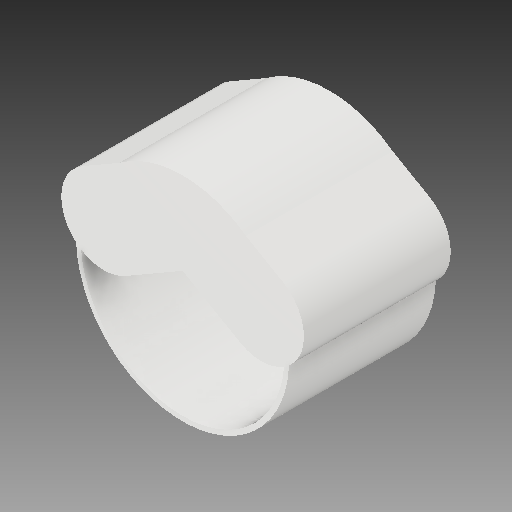
# Autodesk Inventor part: BA001
Saved by Autodesk Inventor 2017 SP1 (Build 210196100, 196)
## iProperties
Created: 2017-06-05
Part Number: BA001
Material: ABS Plastic
Document SubType Name: Modeling
Designer: Zach
Density: 1.06 g/cm^3
Appearance: CR White
Author: Zach
Autodesk Inventor part; units mm, degrees
ref_plane "YZ Plane" through (0, 0, 0) normal (1, 0, 0) x (0, 1, 0)
ref_plane "XZ Plane" through (0, 0, 0) normal (0, 1, 0) x (-1, 0, 0)
ref_plane "XY Plane" through (0, 0, 0) normal (0, 0, 1) x (1, 0, 0)
sketch "Sketch1" plane through (0, 0, 0) normal (0, 0, 1) x (1, 0, 0)
  circle A0 centre (0, 0) radius 225
  dimension "d0" = 450
  constraints: 1 centre point, 1 coincident
  measures "d0" diameter of A0
extrude "Extrusion1" add sketch "Sketch1" along normal blind 10
sketch "Sketch2" plane through (0, 0, 10) normal (0, 0, 1) x (1, 0, 0)
  circle A0 centre (0, 0) radius 225
  circle A1 centre (0, 0) radius 215
  dimension "d3" = 450
  dimension "d4" = 10
  constraints: 2 centre point, 1 coincident
  measures "d3" diameter of A0
  measures "d4" radial gap between concentric circles of A0 A1
extrude "Extrusion2" add sketch "Sketch2" along normal blind 300
sketch "Sketch4" plane through (0, 0, 0) normal (0, 0, 1) x (1, 0, 0)
  circle A0 centre (0, 0) radius 225 construction
  circle A1 centre (-166.2436, 58.2736) radius 90 construction
  circle A2 centre (531.766, -175.9374) radius 90 construction
  line L0 (-90, 206.2159) -> (90, 206.2159) construction
  line L1 (-90, 206.2159) -> (0, 50.3313) construction
  line L2 (-90, 206.2159) -> (90, 206.2159) construction
  line L3 (0, 50.3313) -> (90, 206.2159) construction
  line L4 (-90, 206.2159) -> (-211.2436, 136.2159) construction
  line L5 (0, 50.3313) -> (-121.2436, -19.6687) construction
  line L6 (0, 50.3313) -> (121.2436, -19.6687) construction
  line L7 (90, 206.2159) -> (211.2436, 136.2159) construction
  circle A3 centre (166.2436, 58.2736) radius 90 construction
  arc A4 (-211.2436, 136.2159) -> (-121.2436, -19.6687) centre (-166.2436, 58.2736) ccw
  arc A5 (90, 206.2159) -> (-90, 206.2159) centre (0, 0) ccw
  arc A6 (121.2436, -19.6687) -> (211.2436, 136.2159) centre (166.2436, 58.2736) ccw
  line L8 (-211.2436, 136.2159) -> (-90, 206.2159)
  line L9 (-121.2436, -19.6687) -> (0, 50.3313)
  line L10 (0, 50.3313) -> (121.2436, -19.6687)
  line L11 (90, 206.2159) -> (211.2436, 136.2159)
  dimension "d11" = 450
  dimension "d12" = 180
  dimension "d13" = 180
  dimension "d14" = 180
  dimension "d15" = 180
  dimension "d16" = 60
  dimension "d18" = 140
  dimension "d19" = 140
  dimension "d21" = 90
  dimension "d22" = 90
  dimension "d23" = 140
  dimension "d25" = 90
  dimension "d26" = 140
  dimension "d27" = 90
  dimension "d28" = 180
  constraints: 24 end point, 12 point on circle, 7 centre point, 2 horizontal, 2 tangent, 1 coincident, 1 collinear, 1 concentric, 1 equal length
  measures "d11" diameter of A0
  measures "d12" diameter of A1
  measures "d13" diameter of A2
  measures "d14" distance of L0.start L0.end
  measures "d15" distance of L0.start L1.end
  measures "d16" angle of L1 L2
  measures "d18" distance of L0.start L4.end
  measures "d19" distance of L1.end L5.end
  measures "d21" angle of L1 L4
  measures "d22" angle of L1 L5
  measures "d23" distance of L1.end L6.end
  measures "d25" angle of L6 L3
  measures "d26" distance of L2.end L7.end
  measures "d27" angle of L3 L7
  measures "d28" diameter of A3
extrude "Extrusion4" add sketch "Sketch4" along normal blind 310
body "Solid1"
